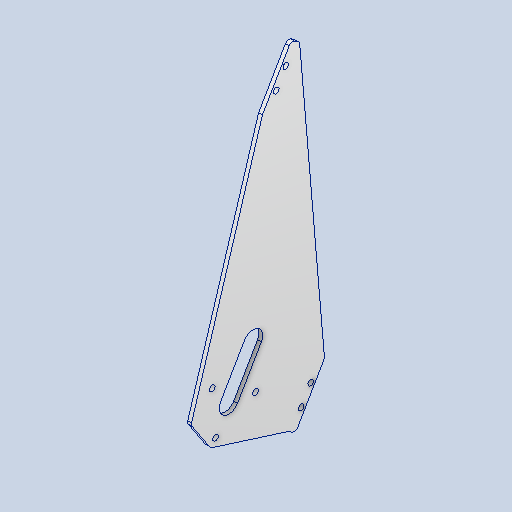
# Autodesk Inventor part: belt_liner_v5_Plate_6
Saved by Autodesk Inventor 2025.2 (Build 292293000, 293)
## iProperties
Created: 2025-02-23
Part Number: belt_liner_v5_Plate_6
Material: アルミニウム 6061
Document SubType Name: Modeling
Designer: haruy
Density: 2.7 g/cm^3
Appearance: アルミニウム - フラット
Author: haruy
Autodesk Inventor part; units mm, degrees
ref_plane "YZ Plane" through (0, 0, 0) normal (1, 0, 0) x (0, 1, 0)
ref_plane "XZ Plane" through (0, 0, 0) normal (0, 1, 0) x (-1, 0, 0)
ref_plane "XY Plane" through (0, 0, 0) normal (0, 0, 1) x (1, 0, 0)
derived "belt_liner_v5_Sketch_Base.ipt"
sketch "スケッチ1" plane through (300, 0, 0) normal (1, 0, 0) x (0, 1, 0)
  circle A0 centre (0, 0) radius 22.36
  circle A1 centre (742.400277, -428.625) radius 23.875 construction
  line L0 (0, 0) -> (0, -985.832038)
  line L1 (0, 0) -> (742.400277, -428.625)
  line L2 (-48.743262, -24.425807) -> (-56.243262, -37.416188)
  line L3 (-56.243262, -37.416188) -> (725.777678, -488.916188)
  line L4 (725.777678, -488.916188) -> (733.277678, -475.925807)
  line L5 (733.277678, -475.925807) -> (-48.743262, -24.425807)
  line L6 (-44.122546, 123.258417) -> (-44.122546, 123.258417)
  line L7 (0, -985.832038) -> (0, 0)
  circle A2 centre (0, 0) radius 12.5
  circle A3 centre (0, 0) radius 15
  line L8 (0, 0) -> (0, 0)
  circle A4 centre (0, 0) radius 24.06 construction
  line L9 (0, 0) -> (0, 0)
  line L10 (0, 0) -> (0, 0)
  line L11 (-48.743262, -24.425807) -> (-46.243262, -20.095679)
  circle A5 centre (742.400277, -428.625) radius 5 construction
  line L12 (733.277678, -475.925807) -> (707.296915, -460.925807)
  line L13 (707.296915, -460.925807) -> (709.796915, -456.595679)
  line L14 (709.796915, -456.595679) -> (735.777678, -471.595679)
  line L15 (735.777678, -471.595679) -> (733.277678, -475.925807)
  circle A6 centre (738.07015, -426.125) radius 5.1
  line L16 (742.400277, -428.625) -> (509.094258, -293.925707)
  circle A7 centre (759.720785, -438.625) radius 5.1
  line L17 (740.62015, -421.70827) -> (762.270785, -434.20827)
  line L18 (735.52015, -430.54173) -> (757.170785, -443.04173)
  circle A8 centre (742.400277, -428.625) radius 22.175 construction
  circle A9 centre (738.07015, -426.125) radius 10.1 construction
  circle A10 centre (759.720785, -438.625) radius 10.1 construction
  line L19 (743.12015, -417.378143) -> (764.770785, -429.878143) construction
  line L20 (733.02015, -434.871857) -> (754.670785, -447.371857) construction
  line L21 (743.12015, -417.378143) -> (730.659838, -410.184179) construction
  line L22 (729.323294, -421.075) -> (734.373294, -412.328143) construction
  line L23 (764.770785, -429.878143) -> (770.933518, -433.436199) construction
  line L24 (770.933518, -433.436199) -> (771.269456, -433.630153)
  line L25 (754.670785, -447.371857) -> (764.770785, -429.878143) construction
  line L26 (764.770785, -429.878143) -> (773.43104, -434.878143)
  line L27 (773.43104, -434.878143) -> (763.33104, -452.371857)
  line L28 (763.33104, -452.371857) -> (754.670785, -447.371857) construction
  circle A11 centre (725.867423, -468.760743) radius 1.5
  circle A12 centre (0, 0) radius 30
  circle A13 centre (742.400277, -428.625) radius 6 construction
  circle A14 centre (0, 0) radius 24.06 construction
  circle A15 centre (0, 0) radius 24.06
  circle A16 centre (742.400277, -428.625) radius 24.06 construction
  line L29 (754.430277, -407.788429) -> (12.03, 20.836571)
  circle A17 centre (725.859192, -419.075) radius 4
  circle A18 centre (725.859192, -419.075) radius 1.5
  circle A19 centre (742.400277, -428.625) radius 18.525 construction
  circle A20 centre (748.98688, -417.41667) radius 4
  line L30 (737.43688, -437.421857) -> (742.48688, -428.675)
  circle A21 centre (748.98688, -417.41667) radius 1.5
  line L31 (734.373294, -412.328143) -> (737.823294, -406.352568) construction
  line L32 (737.823294, -406.352568) -> (776.88104, -428.902568)
  line L33 (773.43104, -434.878143) -> (776.88104, -428.902568)
  line L34 (737.823294, -406.352568) -> (723.650341, -415.740187)
  line L35 (720.823294, -435.797432) -> (759.88104, -458.347432)
  line L36 (720.823294, -435.797432) -> (721.866734, -418.829485)
  line L37 (763.33104, -452.371857) -> (759.88104, -458.347432)
  circle A22 centre (735.98688, -439.93333) radius 4
  circle A23 centre (735.98688, -439.93333) radius 1.5
  circle A24 centre (717.207169, -463.760743) radius 1.5
  circle A25 centre (742.400277, -428.625) radius 34.06
  circle A26 centre (742.48688, -428.675) radius 8.5
  line L38 (-57.983643, -13.420997) -> (-72.983643, -13.420997)
  line L39 (-72.983643, -13.420997) -> (-72.983643, -353.420997)
  line L40 (-72.983643, -353.420997) -> (-57.983643, -353.420997)
  line L41 (-57.983643, -353.420997) -> (-57.983643, -13.420997)
  line L42 (457.016357, -338.420997) -> (-72.983643, -338.420997)
  line L43 (-72.983643, -338.420997) -> (-72.983643, -353.420997)
  line L44 (-72.983643, -353.420997) -> (457.016357, -353.420997)
  line L45 (457.016357, -353.420997) -> (457.016357, -338.420997)
  line L46 (427.016357, -338.420997) -> (427.016357, -353.420997)
  line L47 (457.016357, -353.420997) -> (491.093123, -353.420997)
  line L48 (491.093123, -353.420997) -> (498.593123, -340.430616)
  line L49 (246.77858, -212.365929) -> (254.27858, -199.375548)
  line L50 (-207.983643, 176.579003) -> (-227.983643, 176.579003)
  line L51 (-227.983643, 176.579003) -> (-227.983643, -413.420997)
  line L52 (-227.983643, -413.420997) -> (-207.983643, -413.420997)
  line L53 (-207.983643, -413.420997) -> (-207.983643, 176.579003)
  line L54 (-52.08151, -339.422627) -> (-53.64106, -349.300268)
  line L55 (-53.64106, -349.300268) -> (703.984528, -468.919367)
  line L56 (703.984528, -468.919367) -> (705.544078, -459.041726)
  line L57 (705.544078, -459.041726) -> (-52.08151, -339.422627)
  circle A27 centre (0, 0) radius 24.06
  line L58 (1412.720372, 281.579003) -> (-606.636412, 281.579003)
  line L59 (1185.577585, -518.420997) -> (-909.401992, -518.420997)
  line L60 (9.772119, 46.925807) -> (885.323802, -458.574193)
  line L61 (885.323802, -458.574193) -> (892.823802, -445.583812)
  line L62 (892.823802, -445.583812) -> (17.272119, 59.916188)
  line L63 (17.272119, 59.916188) -> (9.772119, 46.925807)
  line L64 (32.427564, 51.166188) -> (872.472205, -433.833812)
  line L65 (872.472205, -433.833812) -> (876.222205, -427.338622)
  line L66 (876.222205, -427.338622) -> (36.177564, 57.661378)
  line L67 (36.177564, 57.661378) -> (32.427564, 51.166188)
  line L68 (36.177564, 57.661378) -> (94.894086, 23.761378)
  line L69 (94.894086, 23.761378) -> (97.644086, 28.524518)
  line L70 (97.644086, 28.524518) -> (38.927564, 62.424518)
  line L71 (38.927564, 62.424518) -> (36.177564, 57.661378)
  circle A28 centre (215.551935, 104.210607) radius 120
  line L72 (-37.983643, 123.579003) -> (-57.983643, 123.579003)
  line L73 (-57.983643, 123.579003) -> (-57.983643, 103.579003)
  line L74 (-57.983643, 103.579003) -> (-37.983643, 103.579003)
  line L75 (-37.983643, 103.579003) -> (-37.983643, 123.579003)
  line L76 (215.551935, 104.210607) -> (184.493649, 220.121706)
  line L77 (215.551935, 104.210607) -> (99.640835, 73.152321)
  line L78 (215.551935, 104.210607) -> (155.551935, 0.287558)
  line L79 (187.493649, 225.317858) -> (96.640835, 67.956169)
  line L80 (96.640835, 67.956169) -> (91.444683, 70.956169)
  line L81 (91.444683, 70.956169) -> (182.297497, 228.317858)
  line L82 (182.297497, 228.317858) -> (187.493649, 225.317858)
  line L83 (182.297497, 228.317858) -> (179.297497, 223.121706)
  line L84 (179.297497, 223.121706) -> (174.96737, 225.621706)
  line L85 (174.96737, 225.621706) -> (177.96737, 230.817858)
  line L86 (177.96737, 230.817858) -> (182.297497, 228.317858)
  line L87 (91.444683, 70.956169) -> (94.444683, 76.152321)
  line L88 (94.444683, 76.152321) -> (90.114556, 78.652321)
  line L89 (90.114556, 78.652321) -> (87.114556, 73.456169)
  line L90 (87.114556, 73.456169) -> (91.444683, 70.956169)
  line L91 (-37.983643, 123.579003) -> (2.016357, 123.579003)
  line L92 (2.016357, 123.579003) -> (2.016357, 103.579003)
  line L93 (2.016357, 103.579003) -> (-37.983643, 103.579003)
  line L94 (-37.983643, 103.579003) -> (-37.983643, 123.579003)
  circle A29 centre (215.551935, 104.210607) radius 132.068148
  line L95 (101.177564, 170.244681) -> (38.927564, 62.424518)
  line L96 (32.427564, 51.166188) -> (11.695064, 15.256444)
  line L97 (11.695064, 15.256444) -> (20.355318, 10.256444)
  line L98 (20.355318, 10.256444) -> (41.087818, 46.166188)
  line L99 (41.087818, 46.166188) -> (32.427564, 51.166188)
  line L100 (149.517861, -10.163764) -> (155.551935, 0.287558)
  line L101 (149.517861, -10.163764) -> (20.355318, 10.256444)
  line L102 (79.473869, 0.909979) -> (82.973869, 6.972157)
  line L103 (82.973869, 6.972157) -> (98.753155, -2.138017)
  line L104 (179.297497, 223.121706) -> (151.791131, 205.869644)
  line L105 (94.444683, 76.152321) -> (95.632224, 108.599563)
  line L106 (96.640835, 67.956169) -> (113.892897, 40.449803)
  line L107 (-324.983643, 281.579003) -> (-324.983643, -518.420997)
  line L108 (1175.016357, 281.579003) -> (1175.016357, -518.420997)
  line L109 (17.272119, 59.916188) -> (9.772119, 46.925807)
  line L110 (9.772119, 46.925807) -> (-3.218262, 54.425807)
  line L111 (-3.218262, 54.425807) -> (4.281738, 67.416188)
  line L112 (4.281738, 67.416188) -> (17.272119, 59.916188)
  line L113 (-3.218262, 54.425807) -> (-5.718262, 50.095679)
  line L114 (-5.718262, 50.095679) -> (22.427564, 33.845679)
  line L115 (22.427564, 33.845679) -> (24.927564, 38.175807)
  line L116 (24.927564, 38.175807) -> (-3.218262, 54.425807)
  line L117 (-48.743262, -24.425807) -> (-46.243262, -20.095679)
  line L118 (-46.243262, -20.095679) -> (5.718262, -50.095679)
  line L119 (5.718262, -50.095679) -> (3.218262, -54.425807)
  line L120 (3.218262, -54.425807) -> (-48.743262, -24.425807)
  line L121 (789.608636, -403.313017) -> (798.26889, -408.313017)
  line L122 (798.26889, -408.313017) -> (785.03639, -431.232379) construction
  line L123 (785.03639, -431.232379) -> (776.376136, -426.232379)
  line L124 (776.376136, -426.232379) -> (789.608636, -403.313017) construction
  line L125 (885.323802, -458.574193) -> (882.823802, -462.904321)
  line L126 (882.823802, -462.904321) -> (856.84304, -447.904321)
  line L127 (856.84304, -447.904321) -> (859.34304, -443.574193)
  line L128 (859.34304, -443.574193) -> (885.323802, -458.574193)
  line L129 (7.607055, 48.175807) -> (11.937182, 45.675807)
  line L130 (11.937182, 45.675807) -> (19.437182, 58.666188)
  line L131 (19.437182, 58.666188) -> (15.107055, 61.166188)
  line L132 (15.107055, 61.166188) -> (7.607055, 48.175807)
  line L133 (19.437182, 58.666188) -> (14.437182, 50.005934)
  line L134 (14.437182, 50.005934) -> (24.829487, 44.005934)
  line L135 (24.829487, 44.005934) -> (29.829487, 52.666188)
  line L136 (29.829487, 52.666188) -> (19.437182, 58.666188)
  line L137 (931.223149, -485.074193) -> (935.553276, -487.574193)
  line L138 (935.553276, -487.574193) -> (951.553276, -459.861381)
  line L139 (951.553276, -459.861381) -> (947.223149, -457.361381)
  line L140 (947.223149, -457.361381) -> (931.223149, -485.074193)
  line L141 (944.473149, -462.12452) -> (934.973149, -478.579003)
  line L142 (934.973149, -478.579003) -> (919.384691, -469.579003)
  line L143 (919.384691, -469.579003) -> (928.884691, -453.12452)
  line L144 (928.884691, -453.12452) -> (944.473149, -462.12452)
  line L145 (924.134691, -461.351762) -> (939.723149, -470.351762)
  line L146 (926.634691, -457.021635) -> (921.634691, -465.681889)
  line L147 (921.634691, -465.681889) -> (882.663548, -443.181889)
  line L148 (882.663548, -443.181889) -> (887.663548, -434.521635)
  line L149 (887.663548, -434.521635) -> (926.634691, -457.021635)
  line L150 (888.913548, -432.356571) -> (881.413548, -445.346952)
  line L151 (881.413548, -445.346952) -> (874.485345, -441.346952)
  line L152 (874.485345, -441.346952) -> (881.985345, -428.356571)
  line L153 (881.985345, -428.356571) -> (888.913548, -432.356571)
  line L154 (31.079487, 54.831251) -> (23.579487, 41.84087)
  line L155 (23.579487, 41.84087) -> (30.507691, 37.84087)
  line L156 (30.507691, 37.84087) -> (38.007691, 50.831251)
  line L157 (38.007691, 50.831251) -> (31.079487, 54.831251)
  line L158 (16.937182, 54.336061) -> (27.329487, 48.336061)
  circle A30 centre (4.191992, 47.260743) radius 1.25
  circle A31 centre (12.852246, 42.260743) radius 1.25
  line L159 (17.272119, 59.916188) -> (9.772119, 46.925807)
  line L160 (885.323802, -458.574193) -> (882.823802, -462.904321)
  line L161 (882.823802, -462.904321) -> (933.053276, -491.904321)
  line L162 (933.053276, -491.904321) -> (935.553276, -487.574193)
  line L163 (935.553276, -487.574193) -> (885.323802, -458.574193)
  line L164 (375.016357, 281.579003) -> (375.016357, -518.420997)
  line L165 (38.927564, 62.424518) -> (41.427564, 66.754645)
  line L166 (41.427564, 66.754645) -> (100.144086, 32.854645)
  line L167 (100.144086, 32.854645) -> (97.644086, 28.524518)
  line L168 (97.644086, 28.524518) -> (38.927564, 62.424518)
  line L169 (97.724213, 18.663302) -> (115.044721, 8.663302)
  line L170 (115.044721, 8.663302) -> (117.544721, 12.993429)
  line L171 (117.544721, 12.993429) -> (100.224213, 22.993429)
  line L172 (100.224213, 22.993429) -> (97.724213, 18.663302)
  line L173 (116.294721, 10.828365) -> (98.974213, 20.828365)
  line L174 (457.016357, -338.420997) -> (465.112361, -338.420997)
  line L175 (465.112361, -338.420997) -> (472.612361, -325.430616)
  line L176 (-48.743262, -24.425807) -> (-56.243262, -37.416188)
  line L177 (-56.243262, -37.416188) -> (-77.893897, -24.916188)
  line L178 (-77.893897, -24.916188) -> (-70.393897, -11.925807)
  line L179 (-70.393897, -11.925807) -> (-48.743262, -24.425807)
  line L180 (-207.983643, -73.420997) -> (-72.983643, -73.420997)
  line L181 (-72.983643, -73.420997) -> (-72.983643, -93.420997)
  line L182 (-72.983643, -93.420997) -> (-207.983643, -93.420997)
  line L183 (-207.983643, -93.420997) -> (-207.983643, -73.420997)
  line L184 (-72.983643, -273.420997) -> (-207.983643, -273.420997)
  line L185 (-207.983643, -273.420997) -> (-207.983643, -293.420997)
  line L186 (-207.983643, -293.420997) -> (-72.983643, -293.420997)
  line L187 (-72.983643, -293.420997) -> (-72.983643, -273.420997)
  line L188 (-227.983643, -118.420997) -> (-207.983643, -118.420997)
  circle A32 centre (-30.172754, -32.260743) radius 1.25
  circle A33 centre (-12.852246, -42.260743) radius 1.25
  line L189 (-5.718262, 50.095679) -> (-46.243262, -20.095679)
  circle A34 centre (44.676915, 5.382686) radius 15
  circle A35 centre (17.676915, -41.382686) radius 15
  circle A36 centre (44.676915, 5.382686) radius 22
  circle A37 centre (17.676915, -41.382686) radius 22
  circle A38 centre (31.176915, -18) radius 3
  line L190 (44.676915, 5.382686) -> (17.676915, -41.382686)
  circle A39 centre (26.744828, 25.567835) radius 3
  circle A40 centre (-8.769981, -35.945618) radius 3
  circle A41 centre (866.753294, -450.739257) radius 1.25 construction
  circle A42 centre (875.413548, -455.739257) radius 1.25 construction
  line L191 (882.823802, -462.904321) -> (733.277678, -475.925807)
  line L192 (859.34304, -443.574193) -> (737.823294, -406.352568)
  line L193 (722.045397, -417.868779) -> (709.796915, -456.595679)
  circle A43 centre (717.207169, -463.760743) radius 1.5
  circle A44 centre (866.753294, -450.739257) radius 1.5
  circle A45 centre (875.413548, -455.739257) radius 1.5
  circle A46 centre (992.376722, -344.289393) radius 120
  line L194 (275.551935, 208.133655) -> (1052.376722, -240.366345)
  line L195 (-207.983643, -118.420997) -> (1175.016357, -118.420997)
  point P0 (730.659838, -410.184179)
  point P1 (-65.483643, -23.420997)
  point P2 (-65.483643, -345.920997)
  point P3 (447.016357, -345.920997)
  point P4 (437.016357, -345.920997)
  point P5 (477.514285, -336.920997)
  point P6 (486.174539, -341.920997)
  point P7 (-42.983643, -345.920997)
  point P8 (694.886661, -462.420997)
  point P9 (-57.983643, 113.579003)
  point P10 (782.992386, -414.772698)
  point P11 (931.92892, -465.851762)
  dimension "d1" = 3
  dimension "d2" = 3
  dimension "d3" = 3
  measures "d1" diameter of A43
  measures "d2" diameter of A44
  measures "d3" diameter of A45
extrude "押し出し1" add sketch "スケッチ1" against normal blind 2 contours L192 L127 L126 L191 L15 L14 L193 A25 L35 L37 L33 L32 | A25 L32 L192 | A17 L1 A18 | L1 A18 A17 | L193 A17 L36 L35 A25 | L60 L125 L126 L127 | A20 | L32 A25 L33 L27 L37 L35 A22 L30 A26 L18 A7 L17 A6 L1 A17 L34 | A25 L37 L35 | L14 L15 L5 L13 | A17 L1 A6 A26 L30 A22 L35 L36 | A22 | L37 L27 L33 A25 | L32 L33 A25 | A26 A6 L18 L30 | L30 L18 A26 | A26 L17 A6
fillet "フィレット1" radius 2 5 edges at (299, 885.3238, -458.5742) (299, 882.8238, -462.9043) (299, 737.8233, -406.3526) (299, 707.2969, -460.9258) (299, 733.2777, -475.9258)
